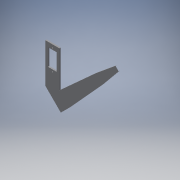
# Autodesk Inventor part: Toe
Saved by Autodesk Inventor 2016 (Build 200138000, 138)
## iProperties
Created: 2015-10-19
Part Number: Toe
Material: Generic
Document SubType Name: Modeling
Designer: powasar16
Density: 1 g/cm^3
Appearance: Default
Author: powasar16
Autodesk Inventor part; units mm, degrees
ref_plane "YZ Plane" through (0, 0, 0) normal (1, 0, 0) x (0, 1, 0)
ref_plane "XZ Plane" through (0, 0, 0) normal (0, 1, 0) x (-1, 0, 0)
ref_plane "XY Plane" through (0, 0, 0) normal (0, 0, 1) x (1, 0, 0)
sketch "Sketch1" plane through (0, 0, 0) normal (0, 0, 1) x (1, 0, 0)
  circle A0 centre (0, -34.925) radius 3.75 projected
  line L0 (-5.9944, -28.9306) -> (5.9944, -28.9306)
  line L1 (5.9944, -28.9306) -> (5.9944, -51.943)
  line L2 (5.9944, -51.943) -> (-5.9944, -51.943)
  line L3 (-5.9944, -51.943) -> (-5.9944, -28.9306)
  line L4 (9.525, -22.5806) -> (-9.525, -22.5806)
  line L5 (-9.525, -22.5806) -> (-9.525, -117.8306)
  line L6 (9.525, -71.8398) -> (9.525, -22.5806)
  line L7 (-9.525, -117.8306) -> (22.9954, -85.3102)
  line L8 (116.1986, 7.893) -> (102.7282, 21.3634) construction
  line L9 (102.7282, 21.3634) -> (72.2546, -9.1102) construction
  line L10 (-5.9944, -39.7604) -> (-9.525, -39.7604) construction
  line L11 (5.9944, -40.4368) -> (9.525, -40.4368) construction
  line L12 (85.725, -22.5806) -> (72.2546, -9.1102) construction
  line L13 (72.2546, -9.1102) -> (9.525, -71.8398) construction
  line L14 (85.725, -22.5806) -> (116.1986, 7.893) construction
  line L15 (67.3489, -36.4666) -> (58.3686, -27.4863) construction
  line L16 (58.3686, -27.4863) -> (56.1235, -25.2413) construction
  line L17 (67.3489, -36.4666) -> (69.5939, -38.7117) construction
  line L18 (9.525, -71.8398) -> (58.3686, -27.4863)
  line L19 (22.9954, -85.3102) -> (67.3489, -36.4666)
  line L20 (22.9954, -85.3102) -> (9.525, -71.8398) construction
  line L21 (67.3489, -36.4666) -> (109.4634, 14.6282)
  line L22 (109.4634, 14.6282) -> (58.3686, -27.4863)
  line L23 (22.9954, -85.3102) -> (85.725, -22.5806) construction
  line L24 (0, -28.9306) -> (0, -22.5806) construction
  dimension "d4" = 5.9944
  dimension "d5" = 5.9944
  dimension "d6" = 11.9888
  dimension "d7" = 23.0124
  dimension "d8" = 19.05
  dimension "d9" = 19.05
  dimension "d10" = 45
  dimension "d11" = 177.8
  dimension "d12" = 95.25
  dimension "d13" = 12.7
  dimension "d14" = 131.8092
  dimension "d15" = 65.9003
  dimension "d18" = 6.35
  constraints: 50 end point, 9 perpendicular, 8 point on line, 7 parallel, 4 midpoint, 2 equal length, 2 horizontal
  measures "d4" distance from line of L1 A0.centre
  measures "d5" distance from line of L0 A0.centre
  measures "d6" distance of L0.start L0.end
  measures "d7" distance between parallel lines of L0 L2
  measures "d8" distance between parallel lines of L5 L6
  measures "d9" distance between parallel lines of L9 L7
  measures "d10" angle of L6 L9
  measures "d11" distance of L5.end L8.start
  measures "d12" distance of L4.end L5.end
  measures "d13" distance of L15.start L15.end
  measures "d14" distance from line of L8 L7.end
  measures "d15" distance from line of L7.end L15
  measures "d18" distance of L24.start L24.end
extrude "Extrusion1" add sketch "Sketch1" along normal blind 1.905 contours L6 L18 L22 L21 L19 L7 L5 L4
sketch "Sketch3" plane through (0, 0, 1.905) normal (0, 0, 1) x (1, 0, 0)
  arc A0 (0.5, -55.291) -> (-0.5, -55.291) centre (0, -54.425) ccw projected
  arc A1 (-0.5, -25.559) -> (0.5, -25.559) centre (0, -26.425) ccw projected
  circle A2 centre (0, -54.425) radius 1
  circle A3 centre (0, -26.425) radius 1
  point P0 (0, 0)
  constraints: 2 centre point, 2 coincident, 2 concentric
extrude "Extrusion2" cut sketch "Sketch3" against normal through all
body "Solid1"
